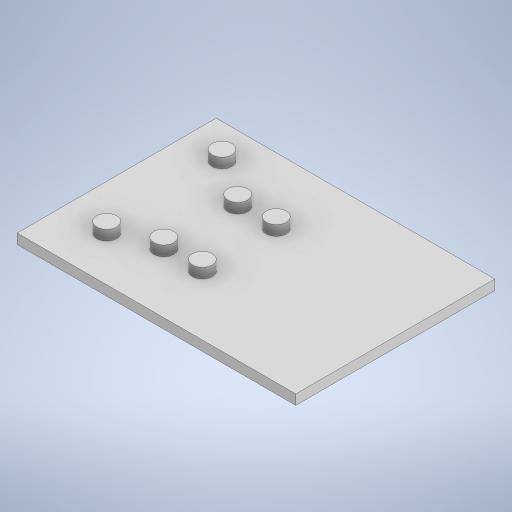
# Autodesk Inventor part: Base
Saved by Autodesk Inventor 2024 (Build 280153000, 153)
## iProperties
Created: 2024-04-22
Part Number: Base
Material: Generic
Document SubType Name: Modeling
Designer: samue
Density: 1 g/cm^3
Appearance: Default
Author: samue
Autodesk Inventor part; units mm, degrees
ref_plane "YZ Plane" through (0, 0, 0) normal (1, 0, 0) x (0, 1, 0)
ref_plane "XZ Plane" through (0, 0, 0) normal (0, 1, 0) x (-1, 0, 0)
ref_plane "XY Plane" through (0, 0, 0) normal (0, 0, 1) x (1, 0, 0)
sketch "Sketch1" plane through (0, 0, 0) normal (0, 1, 0) x (-1, 0, 0)
  line L0 (70, 50) -> (-70, 50)
  line L1 (-70, 50) -> (-70, -50)
  line L2 (-70, -50) -> (70, -50)
  line L3 (70, -50) -> (70, 50)
  line L4 (70, 50) -> (-70, -50) construction
  line L5 (-70, 50) -> (70, -50) construction
  point P0 (0, 0)
  dimension "d0" = 140
  dimension "d1" = 100
  constraints: 12 end point, 2 midpoint, 2 parallel, 1 horizontal, 1 perpendicular
  measures "d0" distance of L2.end L1.end
  measures "d1" distance of L0.end L1.end
extrude "Extrusion1" add sketch "Sketch1" along normal blind 5
sketch "Sketch2" plane through (0, 5, 0) normal (0, 1, 0) x (1, 0, 0)
  circle A0 centre (-50.0251, 32.9196) radius 5
  circle A1 centre (-47.5584, -27.451) radius 5
  circle A2 centre (-26.3779, 17.1894) radius 5
  circle A3 centre (-26.3779, -19.9397) radius 5
  circle A4 centre (-7.0008, 17.1894) radius 5
  circle A5 centre (-7.0008, -19.9397) radius 5
  point P0 (0, 0)
  dimension "d4" = 10
  dimension "d5" = 10
  dimension "d6" = 10
  dimension "d7" = 10
  dimension "d8" = 10
  dimension "d9" = 10
  constraints: 6 centre point
  measures "d4" diameter of A0
  measures "d5" diameter of A1
  measures "d6" diameter of A2
  measures "d7" diameter of A3
  measures "d8" diameter of A4
  measures "d9" diameter of A5
extrude "Extrusion2" add sketch "Sketch2" along normal blind 5
body "Solid1"
